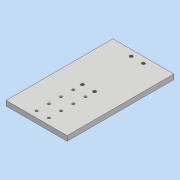
# Autodesk Inventor part: Wspornik pionowy osi Z
Saved by Autodesk Inventor 2018 (Build 220112000, 112)
## iProperties
Created: 2019-01-27
Part Number: Wspornik pionowy osi Z
Material: Ogólny
Document SubType Name: Modeling
Designer: Dawid
Density: 1 g/cm^3
Appearance: Domyślna
Author: Dawid
Autodesk Inventor part; units mm, degrees
ref_plane "YZ Plane" through (0, 0, 0) normal (1, 0, 0) x (0, 1, 0)
ref_plane "XZ Plane" through (0, 0, 0) normal (0, 1, 0) x (-1, 0, 0)
ref_plane "XY Plane" through (0, 0, 0) normal (0, 0, 1) x (1, 0, 0)
sketch "Szkic1" plane through (0, 0, 0) normal (0, 0, 1) x (1, 0, 0)
  line L0 (-50, -65) -> (50, -65)
  line L1 (50, -65) -> (50, 65)
  line L2 (50, 65) -> (-50, 65)
  line L3 (-50, 65) -> (-50, -65)
  line L4 (-50, -65) -> (50, 65) construction
  line L5 (50, -65) -> (-50, 65) construction
  point P0 (0, 0)
  dimension "d0" = 100
  dimension "d1" = 130
  constraints: 12 end point, 2 midpoint, 2 parallel, 1 horizontal, 1 perpendicular
  measures "d0" distance of L2.end L1.end
  measures "d1" distance of L1.end L0.end
extrude "Wyciągnięcie proste1" add sketch "Szkic1" along normal blind 8
sketch "Szkic2" plane through (0, 0, 8) normal (0, 0, 1) x (1, 0, 0)
  line L0 (-16.2, -31.5) -> (-16.2, -58.5)
  line L1 (-16.2, -58.5) -> (16.2, -58.5)
  line L2 (16.2, -31.5) -> (16.2, -58.5)
  line L3 (-16.2, -31.5) -> (16.2, -31.5)
  line L4 (-16.2, -58.5) -> (16.2, -58.5)
  line L5 (16.2, -31.5) -> (-16.2, -58.5)
  line L6 (16.2, -58.5) -> (-16.2, -31.5)
  line L7 (-10, -45) -> (-10, -53.5)
  line L8 (-8.5, -55) -> (8.5, -55)
  line L9 (10, -53.5) -> (10, -36.5)
  line L10 (8.5, -35) -> (-8.5, -35)
  line L11 (-10, -36.5) -> (-10, -45)
  circle A0 centre (10, -55) radius 1.5
  circle A1 centre (-10, -55) radius 1.5
  circle A2 centre (10, -35) radius 1.5
  circle A3 centre (-10, -35) radius 1.5
  line L12 (-50, -65) -> (50, -65) projected
  line L13 (-50, -65) -> (-50, -58.5)
  line L14 (-50, 65) -> (-50, -65) projected
  line L15 (-50, -58.5) -> (50, -58.5)
  line L16 (0, -58.5) -> (0, 0)
  line L17 (0, -45) -> (0, -58.5)
  point P0 (-16.2, -45)
  dimension "d4" = 3
  dimension "d5" = 3
  dimension "d6" = 3
  dimension "d7" = 3
  dimension "d8" = 6.5
  constraints: 32 end point, 8 point on circle, 4 centre point, 4 perpendicular, 3 midpoint, 1 parallel, 1 point on line, 1 vertical
  measures "d4" diameter of A0
  measures "d5" diameter of A1
  measures "d6" diameter of A2
  measures "d7" diameter of A3
  measures "d8" distance of L12.start L13.end
extrude "Wyciągnięcie proste2" cut sketch "Szkic2" against normal up to next contours A3 L6 | L6 A3 | A1 L5 | L5 A1 | A2 L5 | L5 A2 | A0 L6 | L6 A0
sketch "Szkic5" plane through (0, 0, 8) normal (0, 0, 1) x (1, 0, 0)
  line L0 (-16.2, 8.5) -> (-16.2, -18.5)
  line L1 (-16.2, -18.5) -> (16.2, -18.5)
  line L2 (16.2, 8.5) -> (16.2, -18.5)
  line L3 (-16.2, 8.5) -> (16.2, 8.5)
  line L4 (-16.2, -18.5) -> (16.2, -18.5)
  line L5 (16.2, 8.5) -> (-16.2, -18.5)
  line L6 (16.2, -18.5) -> (-16.2, 8.5)
  line L7 (-10, -5) -> (-10, -13.5)
  line L8 (-8.5, -15) -> (8.5, -15)
  line L9 (10, -13.5) -> (10, 3.5)
  line L10 (8.5, 5) -> (-8.5, 5)
  line L11 (-10, 3.5) -> (-10, -5)
  circle A0 centre (10, -15) radius 1.5
  circle A1 centre (-10, -15) radius 1.5
  circle A2 centre (10, 5) radius 1.5
  circle A3 centre (-10, 5) radius 1.5
  line L12 (-50, -65) -> (50, -65)
  line L13 (-50, -65) -> (-50, -58.5)
  line L14 (-50, 65) -> (-50, -65)
  line L15 (-50, -58.5) -> (50, -58.5)
  line L16 (0, -18.5) -> (0, 8.5)
  line L17 (0, -5) -> (0, -18.5)
  line L18 (0, 0) -> (0, -18.5)
  point P0 (-16.2, -5)
  dimension "d15" = 3
  dimension "d16" = 3
  dimension "d17" = 3
  dimension "d18" = 3
  dimension "d19" = 6.5
  dimension "d20" = 18.5
  constraints: 38 end point, 8 point on circle, 4 centre point, 4 perpendicular, 3 midpoint, 2 vertical, 1 parallel, 1 point on line
  measures "d15" diameter of A0
  measures "d16" diameter of A1
  measures "d17" diameter of A2
  measures "d18" diameter of A3
  measures "d19" distance of L12.start L13.end
  measures "d20" distance of L18.start L18.end
extrude "Wyciągnięcie proste5" cut sketch "Szkic5" against normal up to next contours A3 L6 | L6 A3 | A1 L5 | L5 A1 | A2 L5 | L5 A2 | A0 L6 | L6 A0
sketch "Szkic6" plane through (0, 0, 8) normal (0, 0, 1) x (1, 0, 0)
  circle A0 centre (-10, 5) radius 1.5 projected
  circle A1 centre (10, 5) radius 1.5 projected
  circle A2 centre (-10, -15) radius 1.5 projected
  circle A3 centre (10, -35) radius 1.5 projected
  circle A4 centre (-10, -35) radius 1.5 projected
  circle A5 centre (-10, -55) radius 1.5 projected
  circle A6 centre (10, -55) radius 1.5 projected
  circle A7 centre (10, -15) radius 1.5 projected
  point P0 (0, 0)
hole "Otwór1" at (-10, 5, 8) at (10, 5, 8) at (10, -15, 8) at (-10, -15, 8) at (-10, -35, 8) at (10, -35, 8) at (10, -55, 8) at (-10, -55, 8) direction (0, 0, -1) diameter 4 end through all
sketch "Szkic7" plane through (-50, 65, 0) normal (0, 1, 0) x (1, 0, 0)
  line L0 (100, 0) -> (0, 0) projected
  line L1 (0, 0) -> (0, -8) projected
  line L2 (100, -8) -> (0, -8) projected
  line L3 (100, 0) -> (100, -8) projected
  point P0 (50, 0)
extrude "Wyciągnięcie proste6" add sketch "Szkic7" along normal blind 45
sketch "Szkic8" plane through (0, 0, 0) normal (0, 0, -1) x (-1, 0, 0)
  line L0 (-20, 110) -> (-20, 10)
  line L1 (20, 10) -> (-20, 10)
  line L2 (20, 10) -> (20, 110)
  line L3 (-20, 110) -> (20, 110)
  line L4 (-20, 110) -> (20, 10)
  line L5 (20, 110) -> (-20, 10)
  line L6 (0, 0.7274) -> (0, 110)
  line L7 (0, 60) -> (0, 110)
  line L8 (0, 60) -> (0, 10)
  circle A0 centre (-10, 100) radius 2.5
  circle A1 centre (10, 100) radius 2.5
  circle A2 centre (-10, 20) radius 2.5
  circle A3 centre (10, 20) radius 2.5
  line L9 (-50, 110) -> (50, 110) projected
  line L10 (0, 110) -> (0, 109.7979)
  point P0 (0, 0)
  point P1 (-20, 60)
  dimension "d32" = 5
  dimension "d33" = 5
  dimension "d34" = 5
  dimension "d35" = 5
  constraints: 20 end point, 5 midpoint, 4 centre point, 2 vertical
  measures "d32" diameter of A0
  measures "d33" diameter of A1
  measures "d34" diameter of A2
  measures "d35" diameter of A3
extrude "Wyciągnięcie proste7" cut sketch "Szkic8" against normal up to next contours A0 | A1 | A2 | A3
thread "Gwint1" size "M5x0.8" class "6H" standard "ANSI Metric M Profile" full length
thread "Gwint2" size "M5x0.8" class "6H" standard "ANSI Metric M Profile" full length
thread "Gwint3" size "M5x0.8" class "6H" standard "ANSI Metric M Profile" full length
thread "Gwint4" size "M5x0.8" class "6H" standard "ANSI Metric M Profile" full length
